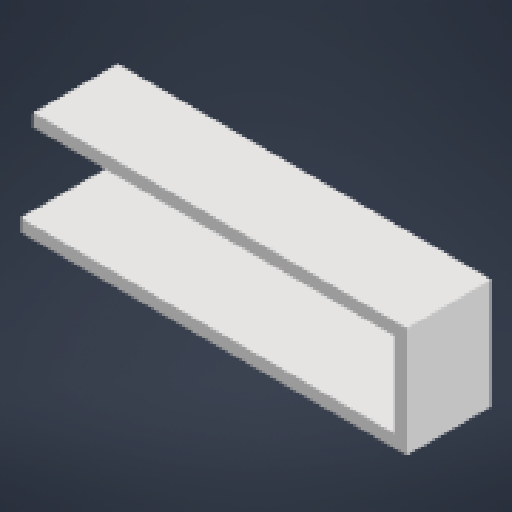
# Autodesk Inventor part: enclosure__bone_bottom
Saved by Autodesk Inventor 2026.2 (Build 302298000, 298)
## iProperties
Created: 2026-04-20
Part Number: enclosure__bone_bottom
Material: Generic
Document SubType Name: Modeling
Designer: Alvin
Density: 1 g/cm^3
Appearance: Default
Author: Alvin
Autodesk Inventor part; units mm, degrees
sketch "Sketch1" plane through (0, 0, 0) normal (0, 1, 0) x (-1, 0, 0)
  line L0 (58.5, 10) -> (-58.5, 10)
  line L1 (-58.5, 10) -> (-58.5, -10)
  line L2 (-58.5, -10) -> (58.5, -10)
  line L3 (58.5, -10) -> (58.5, 10)
  line L4 (58.5, 10) -> (-58.5, -10) construction
  line L5 (-58.5, 10) -> (58.5, -10) construction
  point P0 (0, 0)
  dimension "d0" = 20
  dimension "d1" = 117
  constraints: 12 end point, 2 midpoint, 2 parallel, 1 horizontal, 1 perpendicular
  measures "d0" distance of L2.end L0.start
  measures "d1" distance of L0.start L0.end
extrude "Extrusion1" add sketch "Sketch1" along normal blind 3
sketch "Sketch2" plane through (58.5, 0, 10) normal (1, 0, 0) x (0, 0, -1)
  line L0 (20, 0) -> (20, 3) projected
  line L1 (0, 3) -> (20, 3) projected
  line L2 (0, 0) -> (0, 3) projected
  line L3 (150, -20) -> (0, -20) projected
  line L4 (20, 0) -> (20, -20)
  line L5 (0, 0) -> (0, -20)
  line L6 (20, -20) -> (20, -23)
  line L7 (20, -23) -> (0, -23)
  line L8 (0, -23) -> (0, -20)
  point P0 (10, 0)
  dimension "d4" = 3
  constraints: 10 end point, 3 perpendicular, 1 parallel, 1 point on line, 1 vertical
  measures "d4" distance of L4.end L6.end
extrude "Extrusion2" add sketch "Sketch2" along normal blind 3
sketch "Sketch3" plane through (58.5, -23, -10) normal (0, -1, 0) x (1, 0, 0)
  line L0 (0, 20) -> (0, 0) projected
  line L1 (-120, 20) -> (-120, -3) projected
  line L2 (0, 0) -> (-120, 0)
  line L3 (0, 20) -> (-120, 20)
  point P0 (-58.5, 10)
  constraints: 4 end point, 1 parallel, 1 perpendicular, 1 point on line
ref_plane "Work Plane1" through (-251.5, -20, -8.5) normal (0, -1, 0) x (1, 0, 0)
extrude "Extrusion3" add sketch "Sketch3" against normal up to surface (3 mm away)
move faces "Move1" translate (31.75, 0, 0) faces at (-61.5, -21, 3.3333) (-58.5, 1, -3.3333)
sketch "Sketch4" plane through (-26.75, 0, -10) normal (-1, 0, 0) x (0, 0, 1)
  line L0 (0, 0) -> (20, 0) projected
  line L1 (20, 0) -> (20, 3) projected
  line L2 (0, 3) -> (20, 3) projected
  line L3 (0, 0) -> (0, 3) projected
  point P0 (10, 0)
ref_plane "Work Plane2" through (-57.5, 4, -142) normal (1, 0, 0) x (0, 1, 0)
extrude "Extrusion4" add sketch "Sketch4" along normal up to surface (30.75 mm away)
sketch "Sketch5" plane through (-29.75, -23, -10) normal (-1, 0, 0) x (0, 0, 1)
  line L0 (0, 3) -> (20, 3) projected
  line L1 (0, 0) -> (0, 3) projected
  line L2 (20, 0) -> (0, 0) projected
  line L3 (20, 0) -> (20, 3) projected
  point P0 (10, 23)
ref_plane "Work Plane3" through (-61.5, -23, -141) normal (1, 0, 0) x (0, 1, 0)
extrude "Extrusion5" add sketch "Sketch5" along normal up to surface (31.75 mm away)
sketch "Sketch6" plane through (61.5, -23, -10) normal (0, 0, -1) x (-1, 0, 0)
  line L0 (3, 23) -> (119, 23) projected
  line L1 (119, 26) -> (119, 23) projected
  line L2 (119, 26) -> (0, 26) projected
  line L3 (0, 0) -> (0, 26) projected
  line L4 (123, 0) -> (0, 0) projected
  line L5 (123, 3) -> (123, 0) projected
  line L6 (3, 3) -> (123, 3) projected
  line L7 (3, 3) -> (3, 23) projected
  line L8 (23, 9.4) -> (23, 4.5) projected
  line L9 (23, 0) -> (23, 4.5)
  line L10 (23, 9.4) -> (23, 26)
  point P0 (61.5, 23)
  point P1 (23, 3)
  point P2 (23, 23)
  constraints: 4 end point, 3 point on line, 1 vertical
extrude "Extrusion6" add sketch "Sketch6" along normal blind 65 contours L7 L6 L9 L4 L3 L2 L10 L0
fillet "Fillet1" radius 5 2 edges at (61.5, 3, -32.5) (61.5, -23, -32.5)
sketch "Sketch7" plane through (-61.5, -23, 10) normal (0, -1, 0) x (1, 0, 0)
  circle A0 centre (30.75, -10) radius 2
  line L0 (0, -20) -> (100, -20) projected
  line L1 (0, 0) -> (0, -23) projected
  circle A1 centre (92.25, -10) radius 2
  line L2 (123, -85) -> (123, 0) projected
  point P0 (61.5, -10)
  point P1 (0, -11.5)
  dimension "d0" = 20
  dimension "d1" = 117
  dimension "d19" = 4
  dimension "d20" = 10
  dimension "d21" = 30.75
  dimension "d22" = 4
  dimension "d23" = 10
  dimension "d24" = 30.75
  constraints: 2 centre point, 1 midpoint
  measures "d19" diameter of A0
  measures "d20" distance from line of L0 A0.centre
  measures "d21" horizontal distance of point (0, -11.5) A0.centre
  measures "d22" diameter of A1
  measures "d23" distance from line of A1.centre L0
  measures "d24" distance from line of L2 A1.centre
extrude "Extrusion7" cut sketch "Sketch7" against normal up to surface (26 mm away)
sketch "Sketch8" plane through (61.5, 0, 10) normal (1, 0, 0) x (0, 0, -1)
  line L0 (85, -2) -> (85, -18) projected
  line L1 (0, -2) -> (0, -18) projected
  line L2 (85, -10) -> (0, -10) construction
  circle A0 centre (63.75, -10) radius 2
  circle A1 centre (21.25, -10) radius 2
  line L3 (20, 0) -> (85, 0) projected
  point P0 (10, 0)
  dimension "d27" = 4
  dimension "d28" = 4
  dimension "d29" = 21.25
  dimension "d30" = 21.25
  constraints: 2 centre point, 2 end point, 2 midpoint, 2 point on line
  measures "d27" diameter of A0
  measures "d28" diameter of A1
  measures "d29" distance from line of L1 A1.centre
  measures "d30" distance from line of L0 A0.centre
extrude "Extrusion8" cut sketch "Sketch8" against normal up to surface (3 mm away)
move faces "Move2" translate (0, 0, -65) faces at (59.5, -12.6667, -75)
move faces "Move3" translate (0, 0, -35) faces at (59.5, -10.3208, -55.7241) (59.5, -10.3208, -13.2241)
sketch "Sketch9" plane through (58.5, -20, -140) normal (0, 0, -1) x (-1, 0, 0)
  arc A0 (-3, 2) -> (2, -3) centre (2, 2) ccw projected
  line L0 (2, -3) -> (20, -3) projected
  line L1 (20, -3) -> (20, 0) projected
  line L2 (20, 0) -> (0, 0) projected
  line L3 (0, 0) -> (0, 20) projected
  line L4 (0, 20) -> (20, 20) projected
  line L5 (20, 20) -> (20, 23) projected
  line L6 (20, 23) -> (2, 23) projected
  arc A1 (2, 23) -> (-3, 18) centre (2, 18) ccw projected
  line L7 (-3, 18) -> (-3, 2) projected
  line L8 (0, 20) -> (0, 22.5826)
  line L9 (0, 0) -> (0, -2.5826)
  point P0 (58.5, 20)
  constraints: 4 end point, 2 point on circle, 1 point on line, 1 vertical
ref_plane "Work Plane4" through (-271.5, -18.5, -160) normal (0, 0, -1) x (0, 1, 0)
extrude "Extrusion9" add sketch "Sketch9" along normal up to surface (20 mm away) contours L7 A1 L8 L3 L9 A0 | L9 L2 L1 L0 A0
move faces "Move4" translate (0, 0, -10) faces at (59.5, -11.7321, -87.75) (59.5, -10.3208, -48.2241)
body "Solid1"
